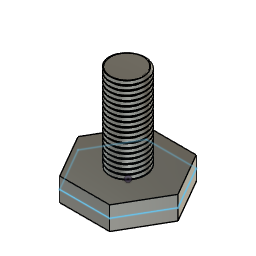
M16Screw (Autodesk Fusion 360 design; units mm, degrees)
Autodesk Fusion 360 part; units mm, degrees
sketch "Sketch1" plane through (0, 0, 0) normal (0, 0, 1) x (1, 0, 0)
  line L0 (-10.9985, 19.05) -> (-21.997, 0)
  line L1 (-21.997, 0) -> (-10.9985, -19.05)
  line L2 (-10.9985, -19.05) -> (10.9985, -19.05)
  line L3 (10.9985, -19.05) -> (21.997, 0)
  line L4 (21.997, 0) -> (10.9985, 19.05)
  line L5 (10.9985, 19.05) -> (-10.9985, 19.05)
  dimension "d8" = 19.05
  measures "d8" distance of origin L2
extrude "Extrude1" add sketch "Sketch1" along normal blind 5.08
sketch "Sketch2" plane through (0, 0, 5.08) normal (0, 0, 1) x (-1, 0, 0)
  line L0 (-10.9985, -19.05) -> (10.9985, -19.05)
  line L1 (10.9985, -19.05) -> (21.997, 0)
  line L2 (21.997, 0) -> (10.9985, 19.05)
  line L3 (10.9985, 19.05) -> (-10.9985, 19.05)
  line L4 (-10.9985, 19.05) -> (-21.997, 0)
  line L5 (-21.997, 0) -> (-10.9985, -19.05)
  circle A0 centre (0, 0) radius 8
  dimension "d3" = 16
  constraint coincident A0.centre origin
  measures "d3" diameter of A0
extrude "Extrude2" add sketch "Sketch2" along normal blind 38.1 contours A0
thread "Thread1" "ANSI Metric M Profile 16.0 M16x2 6g" major diameter 15.822 minor diameter 13.534 pitch 2 angle 60 modelled right hand crest width 0.2847 on face at (-7.9901, 0.3988, 30.48) crest through (-7.911, 0, 4.58)
extrude "Extrude3" add sketch "Sketch1" against normal blind 5.08
